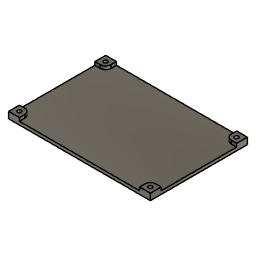
ZesilovacDrzak v3 (Autodesk Fusion 360 design; units mm, degrees)
Autodesk Fusion 360 part; units mm, degrees
sketch "Sketch1" plane through (0, 0, 0) normal (0, 0, 1) x (1, 0, 0)
  circle A0 centre (0, 0) radius 1.8
  circle A1 centre (121.5, 0) radius 1.8
  circle A2 centre (0, 80) radius 1.8
  circle A3 centre (121.5, 80) radius 1.8
  line L0 (-5, -5) -> (126.5, -5)
  line L1 (126.5, -5) -> (126.5, 85)
  line L2 (126.5, 85) -> (-5, 85)
  line L3 (-5, 85) -> (-5, -5)
  dimension "d3" = 121.5
  dimension "d4" = 80
  dimension "d5" = 3.6
  dimension "d6" = 5
  dimension "d7" = 5
  dimension "d8" = 5
  dimension "d9" = 5
  constraint coincident A0.centre origin
  constraint horizontal L0
  constraint vertical L1
  constraint horizontal L2
  constraint vertical L3
  measures "d5" diameter of A0
  measures "d6" horizontal distance of A3.centre L1.end
  measures "d7" distance of A3.centre L2
  measures "d8" vertical distance of A0.centre L0.start
  measures "d9" horizontal distance of A0.centre L0.start
extrude "Extrude1" add sketch "Sketch1" along normal blind 3
sketch "Sketch2" plane through (0, 0, 3) normal (0, 0, 1) x (-1, 0, 0)
  circle A0 centre (0, 0) radius 1.8
  circle A1 centre (0, -80) radius 1.8
  circle A2 centre (-121.5, 0) radius 1.8
  circle A3 centre (-121.5, -80) radius 1.8
  line L0 (5, -85) -> (5, 5)
  line L1 (5, 5) -> (-126.5, 5)
  line L2 (-126.5, 5) -> (-126.5, -85)
  line L3 (-126.5, -85) -> (5, -85)
  circle A4 centre (0, 0) radius 5
  line L4 (-5, 0) -> (-5, 5)
  line L5 (0, -5) -> (5, -5)
  circle A5 centre (-121.5, 0) radius 5
  line L6 (-116.5, 0) -> (-116.5, 5)
  line L7 (-121.5, -5) -> (-126.5, -5)
  circle A6 centre (-121.5, -80) radius 5
  line L8 (-116.5, -80) -> (-116.5, -85)
  line L9 (-121.5, -75) -> (-126.5, -75)
  circle A7 centre (0, -80) radius 5
  line L10 (-5, -80) -> (-5, -85)
  line L11 (0, -75) -> (5, -75)
  constraint concentric A0 A4
  constraint tangent L0 A4
  constraint coincident A4 L4.start
  constraint coincident L1 L4.end
  constraint tangent A4 L4
  constraint perpendicular L1 L4
  constraint coincident A4 L5.start
  constraint coincident L0 L5.end
  constraint tangent A4 L5
  constraint perpendicular L0 L5
  constraint concentric A2 A5
  constraint tangent L1 A5
  constraint coincident A5 L6.start
  constraint coincident L1 L6.end
  constraint tangent A5 L6
  constraint perpendicular L1 L6
  constraint coincident A5 L7.start
  constraint coincident L2 L7.end
  constraint tangent A5 L7
  constraint perpendicular L2 L7
  constraint concentric A3 A6
  constraint tangent L3 A6
  constraint coincident A6 L8.start
  constraint coincident L3 L8.end
  constraint tangent A6 L8
  constraint perpendicular L3 L8
  constraint coincident A6 L9.start
  constraint coincident L2 L9.end
  constraint tangent A6 L9
  constraint perpendicular L2 L9
  constraint concentric A1 A7
  constraint tangent L3 A7
  constraint coincident A7 L10.start
  constraint coincident L3 L10.end
  constraint tangent A7 L10
  constraint perpendicular L3 L10
  constraint coincident A7 L11.start
  constraint coincident L0 L11.end
  constraint tangent A7 L11
  constraint perpendicular L0 L11
extrude "Extrude2" add sketch "Sketch2" along normal blind 3 contours L0 L3 A7 | L0 A7 L11 | A7 | L3 A7 L10 | L0 A4 L5 | L3 A6 L8 | L0 L1 A4 | A4 | L2 L3 A6 | A6 | L1 A4 L4 | L2 A6 L9 | L1 A5 L6 | L2 A5 L7 | L1 L2 A5 | A5
equation "d7 = d6"
equation "d8 = d6"
equation "d9 = d6"
